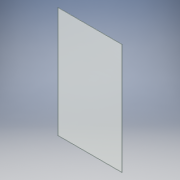
# Autodesk Inventor part: Glass Sheet
Saved by Autodesk Inventor 2017 (Build 210142000, 142)
## iProperties
Created: 2016-09-12
Part Number: Glass Sheet
Material: Glass
Document SubType Name: Modeling
Designer: s.ethan.wierenga
Density: 2.18 g/cm^3
Appearance: Clear
Author: s.ethan.wierenga
Autodesk Inventor part; units mm, degrees
ref_plane "YZ Plane" through (0, 0, 0) normal (1, 0, 0) x (0, 1, 0)
ref_plane "XZ Plane" through (0, 0, 0) normal (0, 1, 0) x (-1, 0, 0)
ref_plane "XY Plane" through (0, 0, 0) normal (0, 0, 1) x (1, 0, 0)
sketch "Sketch1" plane through (0, 0, 0) normal (0, 0, 1) x (1, 0, 0)
  line L0 (0, 0) -> (428.625, 0)
  line L1 (428.625, 0) -> (428.625, 742.95)
  line L2 (428.625, 742.95) -> (0, 742.95)
  line L3 (0, 742.95) -> (0, 0)
  dimension "d0" = 742.95
  dimension "d1" = 428.625
  constraints: 8 end point, 2 parallel, 1 horizontal, 1 perpendicular
  measures "d0" distance of L0.end L1.end
  measures "d1" distance of L0.start L0.end
extrude "Extrusion1" add sketch "Sketch1" along normal blind 3.175
body "Solid1"
